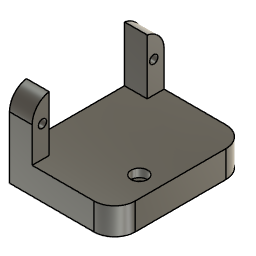
connection v6 (Autodesk Fusion 360 design; units mm, degrees)
Autodesk Fusion 360 part; units mm, degrees
sketch "Sketch1" plane through (0, 0, 0) normal (0, 0, 1) x (1, 0, 0)
  line L0 (31, 32) -> (0, 32)
  line L1 (0, 32) -> (0, 0)
  circle A0 centre (31, 11) radius 2
  line L2 (16, 0) -> (16, 5)
  line L3 (16, 5) -> (0, 5)
  line L4 (31, 32) -> (16, 32)
  line L5 (16, 32) -> (16, 27)
  line L6 (16, 27) -> (0, 27)
  line L7 (31, 32) -> (36, 32)
  line L8 (36, 32) -> (36, 0)
  line L9 (0, 0) -> (36, 0)
  circle A1 centre (31, 11) radius 1
  circle A2 centre (31, 11) radius 2.5
  dimension "d4" = 4
  dimension "d6" = 5
  dimension "d7" = 15
  dimension "d8" = 5
  dimension "d9" = 2
  dimension "d53" = 5
  constraint coincident L1.end L9.start
  constraint coincident L1 L3.end
  constraint perpendicular L1 L3
  constraint perpendicular L4 L5
  constraint coincident L1 L6.end
  constraint perpendicular L1 L6
  constraint horizontal L7
  constraint vertical L8
  constraint perpendicular L8 L9
  constraint concentric A0 A1
  constraint concentric A0 A2
  measures "d4" diameter of A0
  measures "d6" distance of L2.start L2.end
  measures "d7" distance of L0.start L4.end
  measures "d8" distance of L4.end L5.end
  measures "d9" diameter of A1
  measures "d53" diameter of A2
extrude "Extrude1" add sketch "Sketch1" against normal blind 3 contours L0 L1 L2 L3 L4 L5 L6 L7 L8 L9 | L0 L1 L5 L6 | L1 L2 L3 L9
extrude "Extrude2" add sketch "Sketch1" along normal blind 1.5 contours L0 L1 L2 L3 L4 L5 L6 L7 L8 L9 | A0 | A2
sketch "Sketch2" plane through (0, 0, 1.5) normal (0, 0, 1) x (-1, 0, 0)
  circle A0 centre (-31, -11) radius 1
  line L0 (-36, -32) -> (-16, -32)
  line L1 (-16, -32) -> (-16, -27)
  line L2 (-16, -27) -> (0, -27)
  line L3 (0, -27) -> (0, -5)
  line L4 (0, -5) -> (-16, -5)
  line L5 (-16, -5) -> (-16, 0)
  line L6 (-16, 0) -> (-36, 0)
  line L7 (-36, 0) -> (-36, -32)
  circle A1 centre (-31, -11) radius 2
  dimension "d14" = 4
  constraint concentric A0 A1
  measures "d14" diameter of A1
extrude "Extrude3" add sketch "Sketch2" along normal blind 2 contours L0 L1 L2 L3 L4 L5 L6 L7
extrude "Extrude4" add sketch "Sketch1" along normal blind 15.5 contours L0 L1 L5 L6 | L1 L2 L3 L9
sketch "Sketch3" plane through (0, 0, -3) normal (0, 0, -1) x (1, 0, 0)
  line L0 (0, -32) -> (36, -32)
  line L1 (36, -32) -> (36, 0)
  line L2 (36, 0) -> (0, 0)
  line L3 (0, 0) -> (0, -32)
  line L4 (0, 0) -> (-1.5, 0)
  line L5 (-1.5, 0) -> (-1.5, -32)
  line L6 (-1.5, -32) -> (0, -32)
  line L7 (0, -32) -> (0, 0)
  circle A0 centre (31, -11) radius 2.5
  dimension "d19" = 1.5
  constraint horizontal L4
  constraint vertical L5
  constraint horizontal L6
  constraint vertical L7
  constraint coincident L2.end L3.start
  measures "d19" distance of L2.end L4.end
extrude "Extrude5" add sketch "Sketch3" against normal blind 18.5 contours L3 L4 L5 L6 L7
sketch "Sketch4" plane through (0, 0, 15.5) normal (0, 0, 1) x (-1, 0, 0)
  line L0 (-16, -32) -> (1.5, -32)
  line L1 (1.5, -32) -> (1.5, 0)
  line L2 (1.5, 0) -> (-16, 0)
  line L3 (-16, 0) -> (-16, -5)
  line L4 (-16, -5) -> (0, -5)
  line L5 (0, -5) -> (0, -27)
  line L6 (0, -27) -> (-16, -27)
  line L7 (-16, -27) -> (-16, -32)
  line L8 (1.5, 0) -> (-16, 0)
  line L9 (-16, 0) -> (-16, -32)
  line L10 (-16, -32) -> (1.5, -32)
  line L11 (1.5, -32) -> (1.5, 0)
  constraint horizontal L8
  constraint vertical L9
  constraint horizontal L10
  constraint vertical L11
  constraint coincident L0.start L7.end
  constraint coincident L1.end L2.start
extrude "Extrude6" add sketch "Sketch4" along normal blind 1.5
sketch "Sketch5" plane through (16, 0, 0) normal (1, 0, 0) x (0, 1, 0)
  line L0 (0, 3.5) -> (5, 3.5)
  line L1 (5, 3.5) -> (5, 15.5)
  line L2 (5, 15.5) -> (27, 15.5)
  line L3 (27, 15.5) -> (27, 3.5)
  line L4 (27, 3.5) -> (32, 3.5)
  line L5 (32, 3.5) -> (32, 17)
  line L6 (32, 17) -> (0, 17)
  line L7 (0, 17) -> (0, 3.5)
  line L8 (32, 17) -> (32, 11)
  line L9 (32, 11) -> (29.5, 11)
  circle A0 centre (29.5, 11) radius 1
  line L10 (0, 17) -> (0, 11)
  line L11 (0, 11) -> (2.5, 11)
  circle A1 centre (2.5, 11) radius 1
  dimension "d24" = 6
  dimension "d25" = 2.5
  dimension "d26" = 2
  dimension "d27" = 6
  dimension "d28" = 2
  constraint coincident L5.end L6.start
  constraint coincident L5 L8.end
  constraint perpendicular L5 L9
  constraint coincident L9.end A0.centre
  constraint coincident L6.end L7.start
  constraint perpendicular L6 L10
  constraint perpendicular L7 L11
  constraint coincident L11.end A1.centre
  measures "d24" distance of L5.end L8.end
  measures "d25" distance of L8.end L9.end
  measures "d26" diameter of A0
  measures "d27" distance of L6.end L10.end
  measures "d28" diameter of A1
extrude "Extrude7" cut sketch "Sketch5" against normal blind 5 contours A0 | A1
fillet "Fillet1" radius 5 2 edges at (7.25, 0, 17) (7.25, 32, 17)
fillet "Fillet3" radius 5 2 edges at (36, 0, 0.25) (36, 32, 0.25)
sketch "Sketch6" plane through (16, 0, 0) normal (1, 0, 0) x (0, 1, 0)
  arc A0 (32, 12) -> (27, 17) centre (27, 12) ccw
  line L0 (27, 17) -> (5, 17)
  arc A1 (5, 17) -> (0, 12) centre (5, 12) ccw
  line L1 (0, 12) -> (0, 3.5)
  line L2 (0, 3.5) -> (5, 3.5)
  line L3 (5, 3.5) -> (5, 15.5)
  line L4 (5, 15.5) -> (27, 15.5)
  line L5 (27, 15.5) -> (27, 3.5)
  line L6 (27, 3.5) -> (32, 3.5)
  line L7 (32, 3.5) -> (32, 12)
  circle A2 centre (2.5, 11) radius 1
  circle A3 centre (29.5, 11) radius 1
  line L8 (4.5, 15.5) -> (4.5, 3.5)
  line L9 (27.5, 15.5) -> (27.5, 3.5)
  line L10 (4.5, 15.5) -> (4.5, 15.9)
  line L11 (4.5, 15.9) -> (27.5, 15.9)
  line L12 (27.5, 15.9) -> (27.5, 15.5)
  line L13 (4.5, 3.5) -> (27.5, 3.5)
  line L14 (4.5, 15.9) -> (4.5, 16.3)
  line L15 (4.5, 16.3) -> (4.1, 16.3)
  line L16 (27.5, 3.5) -> (27.9, 3.5)
  line L17 (27.9, 3.5) -> (4.1, 3.5)
  line L18 (4.1, 3.5) -> (4.1, 16.3)
  line L19 (4.1, 16.3) -> (27.9, 16.3)
  line L20 (27.9, 16.3) -> (27.9, 3.5)
  line L21 (4.1, 16.3) -> (4.1, 17)
  line L22 (4.1, 17) -> (27.9, 17)
  line L23 (27.9, 17) -> (27.9, 16.3)
  dimension "d37" = 0.5
  dimension "d38" = 0.5
  dimension "d39" = 0.4
  dimension "d48" = 0.4
  dimension "d49" = 0.4
  dimension "d50" = 0.4
  constraint coincident L2 L8.end
  constraint perpendicular L2 L8
  constraint coincident L6 L9.end
  constraint perpendicular L6 L9
  constraint perpendicular L9 L11
  constraint perpendicular L11 L14
  constraint perpendicular L14 L15
  constraint perpendicular L9 L16
  constraint horizontal L17
  constraint vertical L18
  constraint horizontal L19
  constraint vertical L20
  constraint perpendicular L15 L21
  constraint perpendicular L20 L22
  constraint perpendicular L19 L23
  measures "d37" distance of L3.end L8.start
  measures "d38" distance of L4.end L9.start
  measures "d39" distance of L8.start L10.end
  measures "d48" distance of L10.end L14.end
  measures "d49" distance of L14.end L15.end
  measures "d50" distance of L9.end L16.end
extrude "Extrude8" cut sketch "Sketch6" against normal blind 16 contours L6 L9 L11 L12 L14 L16 L17 L19 L20 | L2 L8 L10 L14 L15 L17 L18 L19 | L2 L3 L4 L5 L6 L8 L9 L10 L11 L12 L13 L17
move_face "OffsetFaces1" offset -12 1 faces at (-1.5, 19.6667, 3.6667)
extrude "Extrude10" cut sketch "Sketch6" against normal blind 5.5 contours A0 L0 A1 L15 L19 L21 L22 L23
equation "d17 = 3.50 mm + 12 mm"
